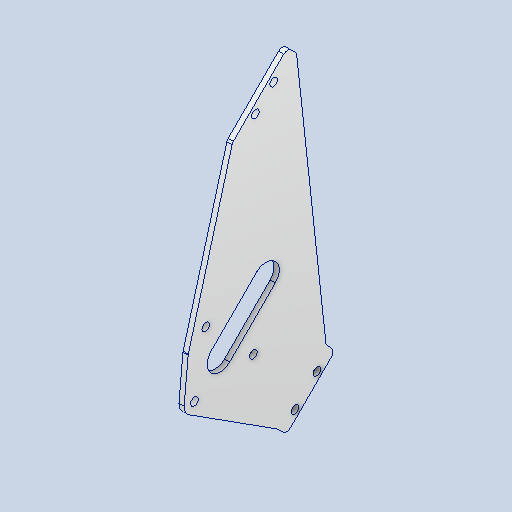
# Autodesk Inventor part: belt_liner_v1_Plate_8
Saved by Autodesk Inventor 2025.2 (Build 292293000, 293)
## iProperties
Created: 2024-12-08
Part Number: belt_liner_v1_Plate_8
Material: アルミニウム 6061
Document SubType Name: Modeling
Designer: haruy
Density: 2.7 g/cm^3
Appearance: アルミニウム - フラット
Author: haruy
Autodesk Inventor part; units mm, degrees
ref_plane "YZ Plane" through (0, 0, 0) normal (1, 0, 0) x (0, 1, 0)
ref_plane "XZ Plane" through (0, 0, 0) normal (0, 1, 0) x (-1, 0, 0)
ref_plane "XY Plane" through (0, 0, 0) normal (0, 0, 1) x (1, 0, 0)
derived "belt_liner_v1_Sketch_Base.ipt"
sketch "スケッチ1" plane through (300, 0, 0) normal (1, 0, 0) x (0, 1, 0)
  circle A0 centre (0, 0) radius 23.875
  circle A1 centre (323.2892, -323.2892) radius 23.875 construction
  line L0 (0, 0) -> (0, -985.832)
  line L1 (14.1421, 50.3106) -> (24.7487, 60.9172)
  line L2 (24.7487, 60.9172) -> (406.5864, -320.9204)
  line L3 (406.5864, -320.9204) -> (395.9798, -331.527)
  line L4 (395.9798, -331.527) -> (14.1421, 50.3106)
  line L5 (0, 0) -> (323.2892, -323.2892)
  line L6 (-50.3106, -14.1421) -> (-60.9172, -24.7487)
  line L7 (-60.9172, -24.7487) -> (289.1006, -374.7666)
  line L8 (289.1006, -374.7666) -> (299.7072, -364.16)
  line L9 (299.7072, -364.16) -> (-50.3106, -14.1421)
  line L10 (22.5524, 63.1136) -> (22.5524, 63.1136)
  line L11 (14.1421, 50.3106) -> (71.3109, -6.8581)
  line L12 (71.3109, -6.8581) -> (67.7754, -10.3937)
  line L13 (67.7754, -10.3937) -> (10.6066, 46.7751)
  line L14 (10.6066, 46.7751) -> (14.1421, 50.3106)
  line L15 (395.9798, -331.527) -> (376.5344, -312.0816)
  line L16 (376.5344, -312.0816) -> (372.9988, -315.6171)
  line L17 (372.9988, -315.6171) -> (392.4443, -335.0625)
  line L18 (392.4443, -335.0625) -> (395.9798, -331.527)
  line L19 (0, -985.832) -> (0, 0)
  circle A2 centre (0, 0) radius 12.5
  circle A3 centre (21.2132, -21.2132) radius 23.5
  circle A4 centre (0, 0) radius 15
  circle A5 centre (21.2132, -21.2132) radius 15
  line L20 (0, 0) -> (0, 0)
  circle A6 centre (-21.2132, 21.2132) radius 15
  circle A7 centre (-21.2132, 21.2132) radius 12.25
  circle A8 centre (0, 0) radius 25.575
  line L21 (0, 0) -> (0, 0)
  line L22 (0, 0) -> (0, 0)
  circle A9 centre (52.7132, -21.2132) radius 1.5
  circle A10 centre (21.2132, -21.2132) radius 31.5
  line L23 (21.2132, -21.2132) -> (49.9041, 7.4777)
  circle A11 centre (21.2132, 10.2868) radius 1.5
  circle A12 centre (-10.2868, -21.2132) radius 1.5
  circle A13 centre (21.2132, -52.7132) radius 1.5
  circle A14 centre (21.2132, -52.7132) radius 3
  circle A15 centre (52.7132, -21.2132) radius 3
  circle A16 centre (21.2132, -52.7132) radius 3
  circle A17 centre (-10.2868, -21.2132) radius 3
  circle A18 centre (21.2132, 10.2868) radius 3
  line L24 (23.3345, 12.4081) -> (54.8345, -19.0919)
  line L25 (54.8345, -23.3345) -> (23.3345, -54.8345)
  line L26 (19.0919, -54.8345) -> (-12.4081, -23.3345)
  line L27 (-50.3106, -14.1421) -> (-46.7751, -10.6066)
  line L28 (-46.7751, -10.6066) -> (10.3937, -67.7754)
  line L29 (10.3937, -67.7754) -> (6.8581, -71.3109)
  line L30 (6.8581, -71.3109) -> (-50.3106, -14.1421)
  line L31 (-15.7223, 32.1636) -> (22.5579, 12.9685)
  line L32 (-32.1636, 15.7223) -> (-12.9685, -22.5579)
  line L33 (84.8528, 0.8132) -> (406.5864, -320.9204)
  line L34 (406.5864, -320.9204) -> (410.4755, -317.0313)
  line L35 (410.4755, -317.0313) -> (88.7419, 4.7023)
  line L36 (88.7419, 4.7023) -> (84.8528, 0.8132)
  circle A19 centre (323.2892, -323.2892) radius 5
  line L37 (299.7072, -364.16) -> (280.9689, -345.4217)
  line L38 (280.9689, -345.4217) -> (284.5044, -341.8861)
  line L39 (284.5044, -341.8861) -> (303.2427, -360.6245)
  line L40 (303.2427, -360.6245) -> (299.7072, -364.16)
  circle A20 centre (319.7537, -319.7537) radius 5.1
  line L41 (323.2892, -323.2892) -> (417.2615, -417.2615)
  circle A21 centre (337.4314, -337.4314) radius 5.1
  line L42 (323.3599, -316.1474) -> (341.0376, -333.8251)
  line L43 (316.1474, -323.3599) -> (333.8251, -341.0376)
  circle A22 centre (323.2892, -323.2892) radius 22.175 construction
  circle A23 centre (323.2892, -323.2892) radius 33.875 construction
  line L44 (374.5443, -310.0916) -> (356.8667, -327.7692)
  line L45 (356.8667, -327.7692) -> (363.9377, -334.8403)
  line L46 (363.9377, -334.8403) -> (381.6154, -317.1626)
  line L47 (381.6154, -317.1626) -> (374.5443, -310.0916)
  circle A24 centre (319.7537, -319.7537) radius 10.1 construction
  circle A25 centre (337.4314, -337.4314) radius 10.1 construction
  line L48 (326.8955, -312.6119) -> (344.5731, -330.2896) construction
  line L49 (312.6119, -326.8955) -> (330.2896, -344.5731) construction
  line L50 (326.8955, -312.6119) -> (318.3599, -304.0764) construction
  line L51 (312.6119, -312.6119) -> (319.7537, -305.4701)
  line L52 (319.7537, -305.4701) -> (376.5344, -312.0816)
  line L53 (392.4443, -335.0625) -> (303.2427, -360.6245)
  line L54 (344.5731, -330.2896) -> (351.3689, -337.0853)
  line L55 (351.3689, -337.0853) -> (351.6442, -337.3606)
  line L56 (71.3109, -6.8581) -> (67.7754, -10.3937)
  line L57 (67.7754, -10.3937) -> (90.8632, -33.4815)
  line L58 (90.8632, -33.4815) -> (94.3988, -29.946)
  line L59 (94.3988, -29.946) -> (71.3109, -6.8581)
  line L60 (244.0828, -334.7487) -> (-45.9172, -334.7487)
  line L61 (-45.9172, -334.7487) -> (-45.9172, -349.7487)
  line L62 (-45.9172, -349.7487) -> (244.0828, -349.7487)
  line L63 (244.0828, -349.7487) -> (244.0828, -334.7487)
  line L64 (-60.9172, -24.7487) -> (-60.9172, -604.2835)
  line L65 (-45.9172, -334.7487) -> (-60.9172, -334.7487)
  line L66 (-60.9172, -334.7487) -> (-60.9172, -349.7487)
  line L67 (-60.9172, -349.7487) -> (-45.9172, -349.7487)
  line L68 (-45.9172, -349.7487) -> (-45.9172, -334.7487)
  line L69 (-60.9172, -334.7487) -> (-45.9172, -334.7487)
  line L70 (-45.9172, -334.7487) -> (-45.9172, -44.7487)
  line L71 (-45.9172, -44.7487) -> (-60.9172, -44.7487)
  line L72 (-60.9172, -44.7487) -> (-60.9172, -334.7487)
  line L73 (330.2896, -344.5731) -> (344.5731, -330.2896) construction
  line L74 (344.5731, -330.2896) -> (351.6442, -337.3606) construction
  line L75 (351.6442, -337.3606) -> (337.3606, -351.6442) construction
  line L76 (337.3606, -351.6442) -> (330.2896, -344.5731)
  line L77 (406.5864, -320.9204) -> (395.9798, -331.527)
  line L78 (395.9798, -331.527) -> (410.1219, -345.6691)
  line L79 (410.1219, -345.6691) -> (420.7285, -335.0625)
  line L80 (420.7285, -335.0625) -> (406.5864, -320.9204)
  line L81 (-12.1904, 2.7649) -> (-50.3106, -35.3553)
  line L82 (-12.1904, 2.7649) -> (35.3553, 50.3106)
  line L83 (6.8581, -71.3109) -> (-3.7485, -81.9175)
  line L84 (-22.0264, -35.3553) -> (-36.1685, -49.4975)
  line L85 (-0.8132, -56.5685) -> (-14.9553, -70.7107)
  circle A26 centre (-30.8652, -30.052) radius 1.5
  circle A27 centre (-13.1875, -47.7297) radius 1.5
  circle A28 centre (2.7224, -63.6396) radius 1.5
  line L86 (49.4975, 36.1685) -> (35.3553, 22.0264)
  line L87 (70.7107, 14.9553) -> (56.5685, 0.8132)
  circle A29 centre (40.6586, 20.2586) radius 1.5
  circle A30 centre (58.3363, 2.5809) radius 1.5
  circle A31 centre (63.6396, -2.7224) radius 1.5
  line L88 (289.4542, -346.8359) -> (285.9186, -350.3714)
  line L89 (297.9394, -355.3212) -> (294.4039, -358.8567)
  circle A32 centre (287.6864, -348.6036) radius 1.5
  circle A33 centre (296.1717, -357.0889) radius 1.5
  line L90 (381.4841, -317.0313) -> (377.9486, -320.5669)
  line L91 (389.9694, -325.5166) -> (386.4339, -329.0521)
  circle A34 centre (379.7163, -318.7991) radius 1.5
  circle A35 centre (388.2016, -327.2844) radius 1.5
  line L92 (284.5044, -341.8861) -> (312.4678, -312.7589)
  line L93 (312.6119, -326.8955) -> (305.4745, -320.0433)
  circle A36 centre (333.8958, -323.1478) radius 1.25
  circle A37 centre (323.1478, -333.8958) radius 1.25
  line L94 (-45.9172, -64.7487) -> (-60.9172, -64.7487)
  line L95 (-10.3106, -54.1421) -> (-20.9172, -64.7487)
  line L96 (-20.9172, -64.7487) -> (-45.9172, -64.7487)
  line L97 (224.0828, -334.7487) -> (224.0828, -349.7487)
  line L98 (244.0828, -349.7487) -> (264.0828, -349.7487)
  line L99 (264.0828, -349.7487) -> (274.6894, -339.1421)
  line L100 (244.0828, -334.7487) -> (249.0828, -334.7487)
  line L101 (249.0828, -334.7487) -> (259.6894, -324.1421)
  line L102 (-45.9172, -44.7487) -> (-40.9172, -44.7487)
  line L103 (-40.9172, -44.7487) -> (-30.3106, -34.1421)
  line L104 (-45.9172, -329.7487) -> (-60.9172, -329.7487)
  line L105 (-25.9172, -334.7487) -> (-25.9172, -349.7487)
  line L106 (-24.8548, -32.5269) -> (-38.9969, -46.669)
  circle A38 centre (0, 0) radius 45
  circle A39 centre (56.9618, -18.8508) radius 22
  circle A40 centre (56.9618, -18.8508) radius 15
  circle A41 centre (79.5495, -33.4815) radius 3
  circle A42 centre (39.0845, -39.0845) radius 3
  circle A43 centre (39.0845, -39.0845) radius 4
  circle A44 centre (18.8508, -56.9618) radius 22
  circle A45 centre (18.8508, -56.9618) radius 15
  circle A46 centre (33.4815, -79.5495) radius 3
  circle A47 centre (39.0845, -39.0845) radius 3
  line L107 (10.3937, -67.7754) -> (6.8581, -71.3109)
  line L108 (6.8581, -71.3109) -> (29.946, -94.3988)
  line L109 (29.946, -94.3988) -> (33.4815, -90.8632)
  line L110 (33.4815, -90.8632) -> (10.3937, -67.7754)
  line L111 (90.8632, -33.4815) -> (33.4815, -90.8632)
  circle A48 centre (76.014, -15.0967) radius 1.5
  circle A49 centre (-20.2586, -40.6586) radius 1.5
  circle A50 centre (-2.5809, -58.3363) radius 1.5
  circle A51 centre (15.0967, -76.014) radius 1.5
  circle A52 centre (323.2892, -323.2892) radius 6
  circle A53 centre (0, 0) radius 25.575 construction
  circle A54 centre (0, 0) radius 25.525
  circle A55 centre (323.2892, -323.2892) radius 25.525 construction
  line L112 (341.3381, -305.2403) -> (18.0489, 18.0489)
  circle A56 centre (309.7835, -309.7835) radius 4
  circle A57 centre (309.7835, -309.7835) radius 1.25 construction
  circle A58 centre (323.2892, -323.2892) radius 18.525 construction
  circle A59 centre (332.5523, -314.1675) radius 4
  line L113 (316.2182, -330.5017) -> (323.3599, -323.3599)
  circle A60 centre (332.5523, -314.1675) radius 1.25 construction
  line L114 (319.7537, -305.4701) -> (324.6327, -300.5911)
  line L115 (324.6327, -300.5911) -> (356.5232, -332.4816) construction
  line L116 (351.6442, -337.3606) -> (356.5232, -332.4816)
  line L117 (324.6327, -300.5911) -> (308.513, -305.9906)
  line L118 (300.5911, -324.6327) -> (332.4816, -356.5232) construction
  line L119 (300.5911, -324.6327) -> (305.9906, -308.513)
  line L120 (337.3606, -351.6442) -> (332.4816, -356.5232)
  circle A61 centre (314.1675, -332.5523) radius 4
  circle A62 centre (314.1675, -332.5523) radius 1.25 construction
  line L121 (376.5344, -312.0816) -> (310.1603, -305.8013)
  line L122 (284.5044, -341.8861) -> (306.4137, -307.6284)
  circle A63 centre (332.5523, -314.1675) radius 1.5
  circle A64 centre (309.7835, -309.7835) radius 1.5
  circle A65 centre (314.1675, -332.5523) radius 1.5
  line L123 (88.7419, 4.7023) -> (131.1683, -37.7241)
  line L124 (131.1683, -37.7241) -> (134.3503, -34.5422)
  line L125 (134.3503, -34.5422) -> (91.9239, 7.8842)
  line L126 (91.9239, 7.8842) -> (88.7419, 4.7023)
  circle A66 centre (258.094, 18.4908) radius 120
  line L127 (134.3503, -34.5422) -> (77.7817, 22.0264)
  line L128 (77.7817, 22.0264) -> (81.3173, 25.5619)
  line L129 (81.3173, 25.5619) -> (137.8858, -31.0066)
  line L130 (137.8858, -31.0066) -> (134.3503, -34.5422)
  line L131 (76.7211, -47.6236) -> (112.0764, -12.2683)
  line L132 (112.0764, -12.2683) -> (119.1475, -19.3394)
  line L133 (119.1475, -19.3394) -> (83.7922, -54.6947)
  line L134 (83.7922, -54.6947) -> (76.7211, -47.6236)
  line L135 (258.094, 18.4908) -> (258.094, 138.4908)
  line L136 (258.094, 18.4908) -> (173.2412, 103.3437)
  line L137 (258.094, 18.4908) -> (138.094, 18.4908)
  line L138 (77.7817, 22.0264) -> (94.3988, -29.946) construction
  circle A67 centre (258.094, 18.4908) radius 130
  line L139 (81.3173, 25.5619) -> (267.9719, 212.2165)
  line L140 (258.094, 138.4908) -> (138.094, 18.4908)
  line L141 (258.094, 138.4908) -> (258.094, 148.4908)
  line L142 (258.094, 18.4908) -> (166.1701, -73.433)
  line L143 (173.2412, -66.362) -> (166.1701, -73.433)
  line L144 (166.1701, -73.433) -> (180.3122, -87.5752)
  line L145 (180.3122, -87.5752) -> (187.3833, -80.5041)
  line L146 (187.3833, -80.5041) -> (173.2412, -66.362)
  line L147 (180.3122, -87.5752) -> (101.4698, -37.017) construction
  line L148 (410.1219, -345.6691) -> (388.9087, -324.4559)
  line L149 (388.9087, -324.4559) -> (385.3732, -327.9915)
  line L150 (385.3732, -327.9915) -> (406.5864, -349.2047)
  line L151 (406.5864, -349.2047) -> (410.1219, -345.6691)
  circle A68 centre (394.212, -333.2948) radius 1.25
  circle A69 centre (401.2831, -340.3658) radius 1.25
  line L152 (120.2082, -20.4) -> (127.2792, -27.4711)
  line L153 (127.2792, -27.4711) -> (91.9239, -62.8264)
  line L154 (91.9239, -62.8264) -> (84.8528, -55.7554)
  line L155 (84.8528, -55.7554) -> (120.2082, -20.4)
  line L156 (104.2983, -36.3099) -> (111.3693, -43.381)
  line L157 (104.2983, -36.3099) -> (77.7817, 22.0264)
  line L158 (111.3693, -43.381) -> (180.3122, -87.5752)
  line L159 (90.8632, -33.4815) -> (94.3988, -29.946)
  line L160 (94.3988, -29.946) -> (102.5305, -38.0777)
  line L161 (102.5305, -38.0777) -> (98.9949, -41.6132)
  line L162 (98.9949, -41.6132) -> (90.8632, -33.4815)
  line L163 (406.5864, -349.2047) -> (303.2427, -360.6245)
  line L164 (319.7537, -305.4701) -> (388.9087, -324.4559)
  line L165 (399.5153, -342.1336) -> (413.6575, -327.9915)
  circle A70 centre (394.212, -333.2948) radius 1.5
  circle A71 centre (401.2831, -340.3658) radius 1.5
  circle A72 centre (86.6206, 16.7231) radius 1.25
  circle A73 centre (93.6916, 9.652) radius 1.25
  circle A74 centre (114.9049, -11.5612) radius 1.25
  circle A75 centre (246.5565, 142.9573) radius 1.5
  line L166 (258.094, 138.4908) -> (138.094, 18.4908)
  line L167 (138.094, 18.4908) -> (145.165, 11.4198)
  line L168 (145.165, 11.4198) -> (265.165, 131.4198)
  line L169 (265.165, 131.4198) -> (258.094, 138.4908)
  line L170 (258.094, 138.4908) -> (248.452, 148.1328)
  line L171 (235.8662, 146.5765) -> (251.0229, 131.4198)
  circle A76 centre (258.094, 18.4908) radius 125
  line L172 (138.094, 18.4908) -> (128.452, 28.1328)
  circle A77 centre (133.6276, 30.0283) radius 1.5
  line L173 (130.0084, 40.7186) -> (145.165, 25.5619)
  point P0 (318.3599, -304.0764)
  point P1 (-53.4172, -334.7487)
  point P2 (287.6864, -348.6036)
  point P3 (345.7281, -331.4446)
  point P4 (345.6734, -331.5937)
  point P5 (344.2037, -330.659)
  point P6 (344.3902, -330.1067)
  point P7 (330.1102, -344.3891)
  point P8 (330.1067, -344.3902)
  point P9 (344.3891, -330.1102)
  point P10 (-53.4172, -49.7487)
  point P11 (-53.4172, -59.7487)
  point P12 (-29.451, -45.6084)
  point P13 (-22.3799, -52.6795)
  point P14 (239.0828, -342.2487)
  point P15 (229.0828, -342.2487)
  point P16 (224.0828, -342.2487)
  point P17 (266.1196, -341.179)
  point P18 (259.0486, -334.108)
  point P19 (-45.9172, -342.2487)
  point P20 (-53.4172, -344.7487)
  point P21 (-53.4172, -334.7487)
  point P22 (-40.9172, -342.2487)
  point P23 (-30.9172, -342.2487)
  point P24 (39.0845, -39.0845)
  point P25 (69.5431, -8.6259)
  point P26 (324.6605, -317.448)
  point P27 (329.1304, -321.9179)
  point P28 (326.6393, -307.3605)
  dimension "d8" = 3
  dimension "d9" = 3
  dimension "d10" = 3
  dimension "d12" = 3
  dimension "d13" = 3
  measures "d8" diameter of A63
  measures "d9" diameter of A64
  measures "d10" diameter of A65
  measures "d12" diameter of A70
  measures "d13" diameter of A71
extrude "押し出し1" add sketch "スケッチ1" along normal blind 2 contours A56 L5 A64 | L5 A64 A56 | A56 L5 A20 L43 A52 A21 L41 L53 L39 L122 | L121 L51 A56 | L39 L88 A32 L9 L38 | L51 L121 L164 L44 L45 L46 L17 L53 L41 A21 L42 A52 A20 L5 | L39 L89 A33 L9 L88 A32 | L39 L40 L9 L89 A33 | L164 L46 L45 L44 | L53 L41 L163 | A52 L42 | L43 L113 A52 | L41 L53 L150 L163 | L43 A52 L113 | L164 L149 L17 | L150 L165 A71 L78 L151 | L18 A70 L17 L91 A35 L4 | L78 L165 A71 L150 L18 A70 | L149 A35 L91 L17 | L4 L91 A35 L149 | A70 L18 A68 | L18 A68 A70 | A35 L91 | A71 L165 A69 | L165 A69 A71 | A35 L91 | A36 | A37 | A59 | A61
fillet "フィレット2" radius 2 8 edges at (301, 303.2427, -360.6245) (301, 299.7072, -364.16) (301, 280.9689, -345.4217) (301, 284.5044, -341.8861) (301, 326.6393, -307.3605) (301, 388.9087, -324.4559) (301, 410.1219, -345.6691) (301, 406.5864, -349.2047)
extrude "押し出し3" cut sketch "スケッチ1" along normal blind 2 contours A70 L18 A68 | L18 A68 A70 | A71 L165 A69 | L165 A69 A71
